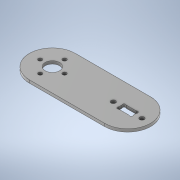
# Autodesk Inventor part: ForeArm_inside_frame_
Saved by Autodesk Inventor 2020.4 (Build 244396000, 396)
## iProperties
Created: 2022-01-10
Part Number: ForeArm_inside_frame_
Material: GFRP
Document SubType Name: Modeling
Designer: Masato Kubotera
Density: 1.75 g/cm^3
Appearance: 滑らか - 標準の灰色
Author: Masato Kubotera
Autodesk Inventor part; units mm, degrees
ref_plane "YZ Plane" through (0, 0, 0) normal (1, 0, 0) x (0, 1, 0)
ref_plane "XZ Plane" through (0, 0, 0) normal (0, 1, 0) x (-1, 0, 0)
ref_plane "XY Plane" through (0, 0, 0) normal (0, 0, 1) x (1, 0, 0)
derived "ForeArm_outside_frame_.ipt"
sketch "スケッチ1" plane through (0, 0, 0) normal (0, 1, 0) x (-1, 0, 0)
  circle A0 centre (0, 0) radius 5.05
  line L0 (0, 8.5) -> (0, -8.5) construction
  circle A1 centre (0, 8.5) radius 1.35
  circle A2 centre (-8.5, 0) radius 1.35
  circle A3 centre (0, -8.5) radius 1.35
  circle A4 centre (8.5, 0) radius 1.35
  circle A5 centre (0, -158.8519) radius 16
  line L1 (0, 0) -> (0, -158.8519) construction
  arc A6 (-16, -121.8654) -> (16, -121.8654) centre (0, -158.8519) ccw
  circle A7 centre (0, 8.5) radius 2.4 construction
  line L2 (-16, 31) -> (16, 31) construction
  line L3 (16, 31) -> (16, -12) construction
  line L4 (16, -12) -> (-16, -12) construction
  line L5 (-16, -12) -> (-16, 31) construction
  line L6 (-16, 31) -> (16, -12) construction
  line L7 (16, 31) -> (-16, -12) construction
  arc A8 (-16, 0) -> (-10.583, -12) centre (0, 0) ccw construction
  arc A9 (10.583, -12) -> (16, 0) centre (0, 0) ccw construction
  line L8 (-16, -121.8654) -> (-16, 0)
  line L9 (16, -121.8654) -> (16, 0)
  circle A10 centre (0, -92.5) radius 1.6
  line L10 (0, -158.8519) -> (-20.1494, -123.952) construction
  circle A11 centre (-17.6494, -128.2822) radius 5 construction
  circle A12 centre (-17.6494, -128.2822) radius 2
  circle A13 centre (-35.2989, -158.8519) radius 2
  circle A14 centre (-17.6494, -189.4216) radius 2
  circle A15 centre (17.6494, -189.4216) radius 2
  circle A16 centre (35.2989, -158.8519) radius 2
  circle A17 centre (17.6494, -128.2822) radius 2
  circle A18 centre (0, -158.8519) radius 58.8961 construction
  line L11 (30.6064, -21.0119) -> (2.8936, -37.0119) construction
  line L12 (2.8936, -37.0119) -> (-18.6064, 0.2272) construction
  line L13 (-18.6064, 0.2272) -> (9.1064, 16.2272) construction
  line L14 (9.1064, 16.2272) -> (30.6064, -21.0119) construction
  line L15 (30.6064, -21.0119) -> (-18.6064, 0.2272) construction
  line L16 (2.8936, -37.0119) -> (9.1064, 16.2272) construction
  line L17 (16.75, -29.0119) -> (-4.75, 8.2272) construction
  circle A19 centre (0, -42.5) radius 1.6
  line L18 (-2.5, -47.5) -> (2.5, -47.5) construction
  line L19 (2.5, -47.5) -> (2.5, -57.5) construction
  line L20 (2.5, -57.5) -> (-2.5, -57.5) construction
  line L21 (-2.5, -57.5) -> (-2.5, -47.5) construction
  line L22 (-2.5, -47.5) -> (2.5, -57.5) construction
  line L23 (2.5, -47.5) -> (-2.5, -57.5) construction
  line L24 (-2.5, -52.5) -> (2.5, -52.5) construction
  circle A20 centre (0, -62.5) radius 1.6
  line L25 (2.8936, -37.0119) -> (54.9285, -127.1389) construction
  line L26 (0, -158.8519) -> (54.9285, -127.1389) construction
  line L27 (-2.5, -47.5) -> (2.5, -47.5) construction
  line L28 (2.5, -47.5) -> (2.5, -87.5) construction
  line L29 (2.5, -87.5) -> (-2.5, -87.5) construction
  line L30 (-2.5, -87.5) -> (-2.5, -47.5) construction
  line L31 (-2.5, -47.5) -> (2.5, -87.5) construction
  line L32 (2.5, -47.5) -> (-2.5, -87.5) construction
  line L33 (-2.55, -47.45) -> (2.55, -47.45)
  line L34 (2.55, -47.45) -> (2.55, -87.55)
  line L35 (2.55, -87.55) -> (-2.55, -87.55)
  line L36 (-2.55, -87.55) -> (-2.55, -47.45)
  line L37 (-2.55, -47.45) -> (2.55, -87.55) construction
  line L38 (2.55, -47.45) -> (-2.55, -87.55) construction
  arc A21 (-1.0651, -47.45) -> (-2.55, -48.9349) centre (-1.8075, -48.1925) ccw
  arc A22 (2.55, -48.9349) -> (1.0651, -47.45) centre (1.8075, -48.1925) ccw
  line L39 (-2.5, -67.5) -> (2.5, -67.5) construction
  arc A23 (-2.55, -86.0651) -> (-1.0651, -87.55) centre (-1.8075, -86.8075) ccw
  arc A24 (1.0651, -87.55) -> (2.55, -86.0651) centre (1.8075, -86.8075) ccw
  arc A25 (16, 0) -> (-16, 0) centre (0, 0) ccw
  circle A26 centre (0, -158.8519) radius 30.2989
  point P0 (0, 9.5)
  point P1 (0, 9.5)
  point P2 (6, -10.3923)
  point P3 (0, -52.5)
  point P4 (0, -67.5)
sketch "スケッチ4" plane through (0, 0, 0) normal (0, 1, 0) x (-1, 0, 0)
  line L0 (-2.55, -87.55) -> (-2.55, -47.45) projected
  line L1 (2.55, -47.45) -> (2.55, -87.55) projected
  line L2 (2.5, -57.5) -> (-2.5, -57.5) construction
  arc A0 (-1.0651, -47.45) -> (-2.55, -48.9349) centre (-1.8075, -48.1925) ccw projected
  arc A1 (2.55, -48.9349) -> (1.0651, -47.45) centre (1.8075, -48.1925) ccw projected
  line L3 (-2.55, -47.45) -> (2.55, -47.45) projected
  line L4 (-2.55, -57.55) -> (2.55, -57.55)
  line L5 (-2.5, -57.5) -> (-2.5, -47.5) construction
  arc A2 (-2.55, -56.0651) -> (-1.0651, -57.55) centre (-1.8075, -56.8075) ccw
  line L6 (0, 0) -> (0, -158.8519) construction
  arc A3 (1.0651, -57.55) -> (2.55, -56.0651) centre (1.8075, -56.8075) ccw
  circle A4 centre (0, -62.5) radius 1.6 projected
  arc A5 (-16, -52.5) -> (16, -52.5) centre (0, -52.5) ccw
  line L7 (-16, -121.8654) -> (-16, 0) projected
  line L8 (16, -121.8654) -> (16, 0) projected
  arc A6 (16, 0) -> (-16, 0) centre (0, 0) ccw projected
  circle A7 centre (0, 8.5) radius 1.35 projected
  circle A8 centre (-8.5, 0) radius 1.35 projected
  circle A9 centre (0, 0) radius 5.05 projected
  circle A10 centre (0, -8.5) radius 1.35 projected
  circle A11 centre (8.5, 0) radius 1.35 projected
  circle A12 centre (0, -42.5) radius 1.6 projected
  point P0 (1.0651, -57.55)
  point P1 (2.55, -56.0651)
  dimension "d6" = 0.05
  dimension "d7" = 0.05
  dimension "d8" = 1.05
  dimension "d9" = 1.05
  dimension "d10" = 10
  constraints: 7 point on circle, 7 point on line, 3 centre point, 3 symmetric about line, 2 end point, 2 tangent, 1 perpendicular, 1 other
  measures "d6" distance between parallel lines of L4 L2
  measures "d7" distance between parallel lines of L0 L5
  measures "d8" radius of A2
  measures "d9" radius of A0
  measures "d10" distance of A4.centre A5.centre
extrude "押し出し2" add sketch "スケッチ4" along normal blind 2 contours A2 L4 A3 L1 A5 L0 | L0 A5 L7 A6 L8 L1 A3 A1 L3 A0 A2
equation "\"d6\" = d7"
equation "\"d8\" = d9"
